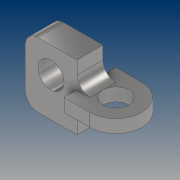
# Autodesk Inventor part: 22
Saved by Autodesk Inventor 2020.2 (Build 242310000, 310)
## iProperties
Created: 2020-09-17
Part Number: 22
Material: 鋼、碳鋼
Document SubType Name: Modeling
Designer: user
Density: 7.85 g/cm^3
Appearance: 半拋光
Mass: 352.138 g
Surface Area: 117.699 cm^2
Volume: 44.8584 cm^3
Author: user
Autodesk Inventor part; units mm, degrees
ref_plane "YZ Plane" through (0, 0, 0) normal (1, 0, 0) x (0, 1, 0)
ref_plane "XZ Plane" through (0, 0, 0) normal (0, 1, 0) x (-1, 0, 0)
sketch "草圖1" plane through (0, 0, 0) normal (0, 0, 1) x (1, 0, 0)
  line L0 (-40, 25) -> (0, 25)
  line L1 (0, 25) -> (0, -25)
  line L2 (0, -25) -> (-40, -25)
  line L3 (-40, -25) -> (-40, 25)
  point P0 (0, 0)
  point P1 (0, 0)
  dimension "d0" = 50
  dimension "d1" = 40
  constraints: 8 end point, 2 parallel, 1 coincident, 1 horizontal, 1 midpoint, 1 perpendicular
  measures "d0" distance of L0.end L1.end
  measures "d1" distance of L0.start L0.end
extrude "擠出1" add sketch "草圖1" along normal mid plane 20
fillet "圓角1" radius 10 2 edges at (-40, 25, 0) (-40, -25, 0)
sketch "草圖2" plane through (0, 0, 10) normal (0, 0, 1) x (1, 0, 0)
  arc A0 (-40, -15) -> (-30, -25) centre (-30, -15) ccw projected
  line L0 (-40, -15) -> (-40, 15) projected
  arc A1 (-30, 25) -> (-40, 15) centre (-30, 15) ccw projected
  line L1 (-30, 25) -> (0, 25) projected
  line L2 (0, 25) -> (0, -25) projected
  line L3 (0, -25) -> (-30, -25) projected
  point P0 (0, 0)
  point P1 (-20, 5)
  dimension "d5" = 20
  dimension "d6" = 20
  measures "d5" distance from line of L1 point (-20, 5)
  measures "d6" distance from line of point (-20, 5) L0
hole "孔1" at (-20, 5, 10) direction (0, 0, -1) diameter 20 end through all
ref_plane "工作平面1" through (0, 0, -10) normal (0, -1, 0) x (1, 0, 0)
sketch "草圖3" plane through (0, 0, -10) normal (0, -1, 0) x (1, 0, 0)
  line L0 (-11.3397, 0) -> (-11.3397, 20) projected
  line L1 (-11.3397, 20) -> (0, 20) projected
  line L2 (0, 20) -> (0, 0) projected
  line L3 (0, 0) -> (-11.3397, 0) projected
  line L4 (-28.6603, 20) -> (-28.6603, 0) projected
  line L5 (-28.6603, 0) -> (-40, 0) projected
  line L6 (-40, 0) -> (-40, 20) projected
  line L7 (-40, 20) -> (-28.6603, 20) projected
  circle A0 centre (20, 10) radius 20
  line L8 (20, -10) -> (0, -10)
  line L9 (0, -10) -> (0, 30)
  line L10 (0, 30) -> (20, 30)
  line L11 (20, 30) -> (20, -10)
  point P0 (0, 10)
  point P1 (0, 10)
  point P2 (20, 10)
  point P3 (0, 20)
  dimension "d15" = 40
  dimension "d14" = 20
  constraints: 8 end point, 2 horizontal, 2 midpoint, 2 parallel, 1 coincident, 1 collinear, 1 horizontal alignment, 1 perpendicular, 3 other
  measures "d14" distance from line of L2 point (20, 10)
extrude "擠出2" add sketch "草圖3" along normal mid plane 10 contours L2 A0 L8 L9 | L9 L10 A0 L2 | A0 L11 | A0 L11
fillet "圓角2" radius 10 2 edges at (0, 5, 0) (0, -5, 0)
sketch "草圖4" plane through (0, 5, -10) normal (0, 1, 0) x (1, 0, 0)
  arc A0 (20, -30) -> (20, 10) centre (20, -10) ccw projected
  point P0 (0, -10)
  constraints: 1 coincident
hole "孔2" at (20, 5, 0) direction (0, -1, 0) diameter 20 end through all
